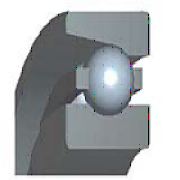
# Autodesk Inventor part: Bearing 1006095 GOST 831-75
Saved by Autodesk Inventor 2018.1 (Build 221171000, 171)
## iProperties
IsCustomPart: 0
Created: 2013-02-12
Part Number: Bearing 1006095 GOST 831-75
Material: Steel, Mild
Description: Single-row angular ball bearings
Document SubType Name: Modeling
Standard: GOST 831-75
Designer: Konstantin
Standards Organization: GOST
Language: en-US
Size Designation: 1006095
Categories: <MemberInstance><Categories><Category DisplayName="Shaft Parts" InternalName="7f7aeb1f-a693-4053-b835-cee3144e0d98" Mnemonic="SHFT"><Category DisplayName="Bearings" InternalName="242d30a3-7172-44e6-a363-b0a3d8f1b556" Mnemonic="BRNG"><CategoryParameter DisplayName="Size Designation" InternalName="2c4e891a-c8f4-49ed-a5c1-5131476c6feb" Mnemonic="sizedes"/><CategoryParameter DisplayName="Shaft Diameter" InternalName="91302473-2833-4451-a660-c5d4a8d6a031" Mnemonic="shaftdia"/><CategoryParameter DisplayName="Outer Diameter" InternalName="d441686c-04bd-4681-b674-94fbc173ec23" Mnemonic="outdia"/><CategoryParameter DisplayName="Width" InternalName="25fc5f6e-338b-4801-b5ed-8959743e396e" Mnemonic="wdth"/><CategoryParameter DisplayName="Basic Dynamic Load Rating" InternalName="440972dd-7009-4861-bd45-69ffbb461423" Mnemonic="bdynlrat"/><CategoryParameter DisplayName="Touch Angle" InternalName="aa21a452-7974-4a55-b5cf-1c2972de2aea" Mnemonic="TouchAngle"/><Category DisplayName="Ball Bearings" InternalName="9b553946-0899-4a5e-a403-c1d9295e77c1" Mnemonic="BALLBEAR"><CategoryParameter DisplayName="Basic Static Load Rating" InternalName="0f13fbbf-c511-4d43-b4c7-197b47424baf" Mnemonic="bstatlrat"/><CategoryParameter DisplayName="Limiting Speed Lubrication Grease" InternalName="5237843b-2c8d-46d3-8227-f3e9dd85a12e" Mnemonic="lubgrsp"/><CategoryParameter DisplayName="Friction Factor" InternalName="3086b0f2-3d69-46ff-8a75-fe12e395bb47" Mnemonic="fricfct"/><CategoryParameter DisplayName="Exponent for Determining Life" InternalName="3029e2ef-9460-4be8-bdfd-dfe61437473d" Mnemonic="lifeexp"/><CategoryParameter DisplayName="Mass" InternalName="7b80f85c-da81-4dea-b8db-d7c689da91b2" Mnemonic="mass"/><CategoryParameter DisplayName="Radius" InternalName="83352640-dfae-4cba-bc9f-11ecbfb0001c" Mnemonic="rad"/><CategoryParameter DisplayName="Min. Shaft Diameter" InternalName="4a5be9bc-ad86-4bf2-8167-102dad5d3e27" Mnemonic="minshaftdia"/><CategoryParameter DisplayName="Max. Hub Step Diameter" InternalName="b5cf89e0-ca87-439c-b08c-a25e2999ab06" Mnemonic="maxhubdia"/><CategoryParameter DisplayName="Max. Step Fillet Radius" InternalName="f6ce6695-cf2c-4ec9-8d20-66671e0e35a4" Mnemonic="maxstprad"/><CategoryParameter DisplayName="Limiting Speed Oil" InternalName="60628548-8907-44dc-8e09-603d72f5766f" Mnemonic="oilspd"/><CategoryParameter DisplayName="Limiting Value for Factor Determination" InternalName="be0ce6fc-cad4-4218-b484-c34dd2571812" Mnemonic="limvalfac"/><CategoryParameter DisplayName="Radial Static Load Factor" InternalName="83ce084d-c51e-4598-a871-e8e1e34b26ee" Mnemonic="raddynfc0"/><CategoryParameter DisplayName="Axial Static Load Factor" InternalName="74dbf5e2-8362-409a-802f-3c2235668d99" Mnemonic="axdynfc0"/><CategoryParameter DisplayName="Radial Dynamic Load Factor when Fa/Fr &lt;= e" InternalName="051e59b3-bd55-4dad-8b07-38b5cb912881" Mnemonic="raddynfc1"/><CategoryParameter DisplayName="Axial Dynamic Load Factor when Fa/Fr &lt;= e" InternalName="ae45a7db-08df-4411-99a8-2f035015bff9" Mnemonic="axdynfc1"/><CategoryParameter DisplayName="Radial Dynamic Load Factor when Fa/Fr &gt; e" InternalName="e513bdb7-139f-4b3c-af32-49e0ba1226b9" Mnemonic="raddynfc2"/><CategoryParameter DisplayName="Axial Dynamic Load Factor when Fa/Fr &gt; e" InternalName="4b6ff741-5956-4a40-80f5-34eb9259f88c" Mnemonic="axdynfc2"/><Category DisplayName="Angular Contact Ball Bearings" InternalName="0b8e5904-7bca-4d33-b75b-fd5460312790" Mnemonic="BBACBB"/></Category></Category></Category><Category DisplayName="DataType" InternalName="23b78d0f-2648-40c6-8793-ca6db495c9e8" Mnemonic="DATATYPE"><CategoryParameter DisplayName="DisplayName" InternalName="05415f3d-3907-474b-a020-eb9d644f4cf3" Mnemonic="DISPLAYNAME"/><CategoryParameter DisplayName="InternalName" InternalName="cf1d0246-76d9-4b4a-8305-fa0409afb5c1" Mnemonic="INTERNALNAME"/><CategoryParameter DisplayName="Folder Name" InternalName="3f06958e-8713-4116-9be7-ed6184ecc97b" Mnemonic="FOLDERNAME"/><CategoryParameter DisplayName="Family Version" InternalName="914462f6-6e19-4b14-ba84-155b9680b1d0" Mnemonic="FAMILYREVISION"/><CategoryParameter DisplayName="ClipFormat" InternalName="bc51e27b-3422-4e78-93ef-cec197ddf230" Mnemonic="CLIPFORMAT"/><CategoryParameter DisplayName="IsMetric" InternalName="e2385c5b-1ea4-4823-96a8-8de651266ec3" Mnemonic="ISMETRIC"/><CategoryParameter DisplayName="Description" InternalName="13903e3d-64b1-4950-80da-f627842ea37f" Mnemonic="DESCRIPTION"/><CategoryParameter DisplayName="StdsOrg" InternalName="8f5914e1-4693-403f-8ab5-d37768198c9d" Mnemonic="STDSORG"/><CategoryParameter DisplayName="Standard" InternalName="0c0a119c-1e12-4c84-803f-101930972f5e" Mnemonic="STANDARD"/><CategoryParameter DisplayName="Manufacturer" InternalName="cd6c7a72-a28a-4e50-99a9-2c7f4e13e5ad" Mnemonic="MANUFACTURER"/><CategoryParameter DisplayName="Member Revision" InternalName="a65d44b9-392f-4f4f-857b-e4b3d54996fe" Mnemonic="MEMBERREVISION"/><CategoryParameter DisplayName="Standard Revision" InternalName="91d5a463-65c2-4fde-b823-3b7fea5e8e17" Mnemonic="STANDARDREVISION"/><CategoryParameter DisplayName="Revision Guid" InternalName="45a75005-10b1-4dfc-8d6d-dfe629f0b93c" Mnemonic="REVISIONGUID"/><CategoryParameter DisplayName="Designation" InternalName="2675968c-4ce5-49e0-a4f5-552d29089031" Mnemonic="DESIGNATION"/><CategoryParameter DisplayName="FileName" InternalName="8b46a4cc-9585-4fed-90c3-899f57e09a73" Mnemonic="FILENAME"/><CategoryParameter DisplayName="Default Row" InternalName="2af9ec52-faaa-4026-b378-f9fa4afca842" Mnemonic="DEFAULTROW"/><Category DisplayName="Part" InternalName="c0e0b642-3bcb-4cc8-9e80-f96d35c4afa4" Mnemonic="PART"><CategoryParameter DisplayName="Material" InternalName="818a152a-d3c3-49ca-80ee-df7d91421b8e" Mnemonic="MATERIAL"/><CategoryParameter DisplayName="Material Key" InternalName="5c9a8adb-dd2b-4535-b97f-0a94a95fe41f" Mnemonic="MATERIALKEY"/><CategoryParameter DisplayName="Part Number" InternalName="016b6077-bfbe-49bd-92c9-d8d59c39c941" Mnemonic="PARTNUMBER"/><CategoryParameter DisplayName="Stock Number" InternalName="4dba7c1c-e26c-444e-836c-b08b433409a8" Mnemonic="STOCKNUMBER"/></Category></Category></Categories><FamilyTemplate Id="Bearing 6000 GOST 831-75"><FamilyTemplateParameters><FamilyTemplateParameter ObjectType="kUserParameterObject" ValueType="xs:double" Id="1" ObjectReferenceKey="a"/><FamilyTemplateParameter ObjectType="kUserParameterObject" ValueType="xs:double" Id="2" ObjectReferenceKey="B"/><FamilyTemplateParameter ObjectType="kUserParameterObject" ValueType="xs:double" Id="3" ObjectReferenceKey="C0"/><FamilyTemplateParameter ObjectType="kUserParameterObject" ValueType="xs:double" Id="4" ObjectReferenceKey="C_"/><FamilyTemplateParameter ObjectType="kUserParameterObject" ValueType="xs:double" Id="5" ObjectReferenceKey="D"/><FamilyTemplateParameter ObjectType="kUserParameterObject" ValueType="xs:double" Id="6" ObjectReferenceKey="d_"/><FamilyTemplateParameter ObjectType="kUserParameterObject" ValueType="xs:double" Id="8" ObjectReferenceKey="r"/><FamilyTemplateParameter ObjectType="kUserParameterObject" ValueType="xs:double" Id="9" ObjectReferenceKey="r1"/><FamilyTemplateParameter ObjectType="kPropertyObject" ValueType="xs:string" Id="100" ObjectReferenceKey="{32853F0F-3444-11d1-9E93-0060B03C1CA6}" SubObjectId="52"/><FamilyTemplateParameter ObjectType="kPropertyObject" ValueType="xs:string" Id="105" ObjectReferenceKey="{32853F0F-3444-11d1-9E93-0060B03C1CA6}" SubObjectId="5"/><FamilyTemplateParameter ObjectType="kPartComponentDefinitionObject" ValueType="xs:string" Id="110" SubObjectId="Material"/></FamilyTemplateParameters></FamilyTemplate><CategoryParameterMap><ParamToTemplateMap><ParamToTemplate CategoryParameter="//CategoryParameter[@InternalName='05415f3d-3907-474b-a020-eb9d644f4cf3']" ConstantValue="Bearing 6000 GOST 831-75"/><ParamToTemplate CategoryParameter="//CategoryParameter[@InternalName='0c0a119c-1e12-4c84-803f-101930972f5e']" ConstantValue="GOST 831-75"/><ParamToTemplate CategoryParameter="//CategoryParameter[@InternalName='13903e3d-64b1-4950-80da-f627842ea37f']" ConstantValue="Single-row angular ball bearings"/><ParamToTemplate CategoryParameter="//CategoryParameter[@InternalName='2af9ec52-faaa-4026-b378-f9fa4afca842']" ConstantValue="1"/><ParamToTemplate CategoryParameter="//CategoryParameter[@InternalName='3f06958e-8713-4116-9be7-ed6184ecc97b']" ConstantValue="Bearing 6000 GOST 831-75"/><ParamToTemplate CategoryParameter="//CategoryParameter[@InternalName='45a75005-10b1-4dfc-8d6d-dfe629f0b93c']" ConstantValue="086c5168-591d-4309-961d-8c724c363079"/><ParamToTemplate CategoryParameter="//CategoryParameter[@InternalName='8f5914e1-4693-403f-8ab5-d37768198c9d']" ConstantValue="GOST"/><ParamToTemplate CategoryParameter="//CategoryParameter[@InternalName='914462f6-6e19-4b14-ba84-155b9680b1d0']" ConstantValue="11"/><ParamToTemplate CategoryParameter="//CategoryParameter[@InternalName='91d5a463-65c2-4fde-b823-3b7fea5e8e17']" TemplateParameter="103"/><ParamToTemplate CategoryParameter="//CategoryParameter[@InternalName='bc51e27b-3422-4e78-93ef-cec197ddf230']" ConstantValue="CF_INVENTOR.STDPARTS"/><ParamToTemplate CategoryParameter="//CategoryParameter[@InternalName='cd6c7a72-a28a-4e50-99a9-2c7f4e13e5ad']" TemplateParameter="104"/><ParamToTemplate CategoryParameter="//CategoryParameter[@InternalName='cf1d0246-76d9-4b4a-8305-fa0409afb5c1']" ConstantValue="07ed72d2-44f7-45dd-8c35-531f6f3084be"/><ParamToTemplate CategoryParameter="//CategoryParameter[@InternalName='e2385c5b-1ea4-4823-96a8-8de651266ec3']" ConstantValue="true"/><ParamToTemplate CategoryParameter="//CategoryParameter[@InternalName='8b46a4cc-9585-4fed-90c3-899f57e09a73']" ConstantValue="Bearing 1006095 GOST 831-75"/><ParamToTemplate CategoryParameter="//CategoryParameter[@InternalName='a65d44b9-392f-4f4f-857b-e4b3d54996fe']" ConstantValue="42341cc5-4857-4ab2-949a-cdbb552f0a97"/><ParamToTemplate CategoryParameter="//CategoryParameter[@InternalName='25fc5f6e-338b-4801-b5ed-8959743e396e']" TemplateParameter="2"/><ParamToTemplate CategoryParameter="//CategoryParameter[@InternalName='d441686c-04bd-4681-b674-94fbc173ec23']" TemplateParameter="5"/><ParamToTemplate CategoryParameter="//CategoryParameter[@InternalName='2675968c-4ce5-49e0-a4f5-552d29089031']" TemplateParameter="100"/><ParamToTemplate CategoryParameter="//CategoryParameter[@InternalName='2c4e891a-c8f4-49ed-a5c1-5131476c6feb']" TemplateParameter="100"/><ParamToTemplate CategoryParameter="//CategoryParameter[@InternalName='818a152a-d3c3-49ca-80ee-df7d91421b8e']" TemplateParameter="110"/><ParamToTemplate CategoryParameter="//CategoryParameter[@InternalName='016b6077-bfbe-49bd-92c9-d8d59c39c941']" TemplateParameter="105"/><ParamToTemplate CategoryParameter="//CategoryParameter[@InternalName='91302473-2833-4451-a660-c5d4a8d6a031']" TemplateParameter="6"/></ParamToTemplateMap></CategoryParameterMap></MemberInstance>
Mass: 2.50305 g
Surface Area: 7.57755 cm^2
Volume: 0.318454 cm^3
Density: 7.86 g/cm^3
Appearance: Steel
Title: Подшипник
Author: Konstantin
Autodesk Inventor part; units mm, degrees
ref_plane "YZ Plane" through (0, 0, 0) normal (1, 0, 0) x (0, 1, 0)
ref_plane "XZ Plane" through (0, 0, 0) normal (0, 1, 0) x (-1, 0, 0)
ref_plane "XY Plane" through (0, 0, 0) normal (0, 0, 1) x (1, 0, 0)
sketch "Sketch1" plane through (0, 0, 0) normal (0, 0, 1) x (1, 0, 0)
  line L0 (0, 6.1) -> (0, 5.3)
  line L1 (4, 5.1667) -> (4, 6.3)
  line L2 (3.8, 6.5) -> (0.4, 6.5)
  line L3 (4, 3.7) -> (4, 2.9)
  line L4 (3.6, 2.5) -> (0.4, 2.5)
  line L5 (0, 2.9) -> (0, 3.7)
  circle A0 centre (2, 4.5) radius 0.8889
  line L6 (0.1333, 5.1667) -> (1.4121, 5.1667)
  line L7 (2.5879, 5.1667) -> (4, 5.1667)
  line L8 (0.1333, 3.8333) -> (1.4121, 3.8333)
  line L9 (2.5879, 3.8333) -> (3.8667, 3.8333)
  line L10 (-0.378, 0) -> (1.978, 0) projected
  line L11 (2, 5.3889) -> (3.294, 5.6639)
  line L12 (2, 2.5) -> (2, 6.5)
  line L13 (3.294, 5.6639) -> (3.4273, 5.7973)
  arc A1 (0.4, 6.5) -> (0, 6.1) centre (0.4, 6.1) ccw
  arc A2 (3.6, 2.5) -> (4, 2.9) centre (3.6, 2.9) ccw
  arc A3 (0, 2.9) -> (0.4, 2.5) centre (0.4, 2.9) ccw
  arc A4 (4, 6.3) -> (3.8, 6.5) centre (3.8, 6.3) ccw
  line L14 (3.4273, 5.7973) -> (3.8667, 5.7973)
  line L15 (3.8667, 5.7973) -> (4, 5.9306)
  line L16 (0, 5.3) -> (0.1333, 5.1667)
  line L17 (0.1333, 3.8333) -> (0, 3.7)
  line L18 (3.8667, 3.8333) -> (4, 3.7)
  line L19 (0.8444, 4.8333) -> (3.1556, 4.8333)
  line L20 (3.1556, 4.8333) -> (3.1556, 4.1667)
  line L21 (3.1556, 4.1667) -> (0.8444, 4.1667)
  line L22 (0.8444, 4.1667) -> (0.8444, 4.8333)
  point P0 (0, 0)
  point P1 (0, 5.1667)
  point P2 (0, 3.8333)
  point P3 (4, 3.8333)
  point P4 (3.294, 5.1667)
  point P5 (2, 3.6111)
  point P6 (2, 4.8333)
  point P7 (0.8444, 4.5)
  dimension "d1" = 1.7778
  dimension "d0" = 5
  dimension "d2" = 13
  dimension "d3" = 4
  dimension "d4" = 1.3333
  dimension "d5" = 12
  dimension "d6" = 0.4
  dimension "d7" = 0.2
  dimension "d8" = 45
  dimension "d9" = 0.1333
  dimension "d10" = 0.1333
  dimension "d11" = 0.1333
  dimension "d12" = 0.1333
  dimension "d13" = 0.1333
  dimension "d14" = 0.1333
  dimension "d15" = 0.1333
  dimension "d17" = 0.6667
  dimension "d18" = 2.3111
  constraints: 44 end point, 14 point on line, 11 parallel, 8 point on circle, 8 tangent, 7 perpendicular, 5 midpoint, 4 centre point, 3 collinear, 2 equal length, 2 equal radius, 2 vertical alignment, 1 coincident, 1 horizontal, 1 horizontal alignment, 1 vertical, 9 other
  measures "d0" diameter of L4 L10
  measures "d2" diameter of L2 L10
  measures "d3" distance between parallel lines of L3 L5
  measures "d4" distance between parallel lines of L4 L9
  measures "d5" angle of L7 L11
  measures "d6" radius of A1
  measures "d7" radius of A4
  measures "d8" angle of L7 L13
  measures "d9" distance from line of L14 L11.end
  measures "d10" distance of L0.end point (0, 5.167)
  measures "d11" distance of L6.start point (0, 5.167)
  measures "d12" distance of L8.start point (0, 3.833)
  measures "d13" distance of L5.end point (0, 3.833)
  measures "d14" distance of L9.end point (4, 3.833)
  measures "d15" distance of L3.start point (4, 3.833)
  measures "d17" distance between parallel lines of L21 L19
  measures "d18" distance between parallel lines of L20 L22
revolve "Revolution1" add sketch "Sketch1" angle 360 about axis through (-10, 0, 0) along (1, 0, 0) contours A1 L2 L12 A0 L6 L16 L0 | L2 A4 L1 L15 L14 L13 L11 L12 | L19 L12 L21 A0 | A0 L21 L22 L19 | L19 A0 L21 L12 | L19 L20 L21 A0 | A0 L12 L4 A3 L5 L17 L8 | A0 L9 L18 L3 A2 L4 L12
revolve "Revolution2" add sketch "Sketch1" angle 360 about axis through (2, 2.5, 0) along (0, 1, 0) picked at (2.3333, 5.0959) picked at (2.2963, 4.5) picked at (2.3333, 3.9041) contours A0 L19 L12 | L19 A0 L21 L12 | L21 A0 L12
pattern_circular "Circular Pattern1" count 11 over 360 about axis through (1.2, 0, 0) along (1, 0, 0) of "Revolution2"
equation "\"d1\" = -0.222222 * d_ + 0.222222 * D"
equation "\"d0\" = d_"
equation "\"d2\" = D"
equation "\"d3\" = B"
equation "\"d4\" = -0.166667 * d_ + 0.166667 * D"
equation "\"d5\" = a"
equation "\"d6\" = r"
equation "\"d7\" = r1"
equation "\"d9\" = 0.1 * d4"
equation "\"d10\" = 0.333333 * r"
equation "\"d11\" = d10"
equation "\"d12\" = d10"
equation "\"d13\" = d12"
equation "\"d14\" = d10"
equation "\"d15\" = d14"
equation "\"d17\" = 0.5 * d4"
equation "\"d18\" = 1.3 * d1"
equation "\"d_\" = 5"
equation "\"D\" = 13"
equation "\"B\" = 4"
equation "\"r\" = 0.4"
equation "\"r1\" = 0.2"
equation "\"a\" = 12deg"
body "Solid1"
